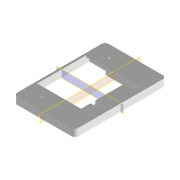
# Autodesk Inventor part: TIRFImager_base_v0
Saved by Autodesk Inventor 2022 (Build 260153000, 153)
## iProperties
Created: 2022-05-21
Part Number: TIRFImager_base_v0
Material: Generisch
Document SubType Name: Modeling
Designer: diederichbenedict
Density: 1 g/cm^3
Appearance: Vorgabe
Author: diederichbenedict
Autodesk Inventor part; units mm, degrees
ref_plane "YZ Plane" through (0, 0, 0) normal (1, 0, 0) x (0, 1, 0)
ref_plane "XZ Plane" through (0, 0, 0) normal (0, 1, 0) x (-1, 0, 0)
ref_plane "XY Plane" through (0, 0, 0) normal (0, 0, 1) x (1, 0, 0)
sketch "Skizze1" plane through (0, 0, 0) normal (0, 1, 0) x (-1, 0, 0)
  line L0 (-37.75, -63.9) -> (37.75, -63.9)
  line L1 (42.75, -58.9) -> (42.75, 58.9)
  line L2 (37.75, 63.9) -> (-37.75, 63.9)
  line L3 (-42.75, 58.9) -> (-42.75, -58.9)
  line L4 (-42.75, -63.9) -> (42.75, 63.9) construction
  line L5 (42.75, -63.9) -> (-42.75, 63.9) construction
  arc A0 (42.75, 58.9) -> (37.75, 63.9) centre (37.75, 58.9) ccw
  arc A1 (-37.75, 63.9) -> (-42.75, 58.9) centre (-37.75, 58.9) ccw
  arc A2 (-42.75, -58.9) -> (-37.75, -63.9) centre (-37.75, -58.9) ccw
  arc A3 (37.75, -63.9) -> (42.75, -58.9) centre (37.75, -58.9) ccw
  point P0 (0, 0)
  dimension "d0" = 85.5
  dimension "d1" = 127.8
  dimension "d2" = 5
  constraints: 12 end point, 8 point on circle, 8 point on line, 8 tangent, 4 centre point, 3 equal radius, 2 midpoint, 2 parallel, 1 horizontal, 1 perpendicular
  measures "d0" distance of L5.end L4.end
  measures "d1" distance of L4.end L5.start
  measures "d2" radius of A0
extrude "Extrusion1" add sketch "Skizze1" along normal blind 10
ref_plane "Arbeitsebene1" through (37.75, 0, 0) normal (0, 0, -1) x (-1, 0, 0)
ref_plane "Arbeitsebene2" through (0, 0, 58.9) normal (1, 0, 0) x (0, 0, -1)
sketch "Skizze2" plane through (0, 10, 0) normal (0, 1, 0) x (1, 0, 0)
  line L0 (-12.95, 38) -> (-38.75, 38) projected
  line L1 (-38.75, -38) -> (-12.95, -38) projected
  line L2 (-12.95, -38) -> (-12.95, -2.5) projected
  line L3 (-38.75, 38) -> (-38.75, -38) projected
  line L4 (-38.75, -38) -> (-12.95, -38)
  line L5 (-12.95, -38) -> (-12.95, 38)
  line L6 (-12.95, 38) -> (-38.75, 38)
  line L7 (-38.75, 38) -> (-38.75, -38)
  line L8 (-11.95, 39) -> (-11.95, -39)
  line L9 (-11.95, -39) -> (-39.75, -39)
  line L10 (-39.75, -39) -> (-39.75, 39)
  line L11 (-39.75, 39) -> (-11.95, 39)
  point P0 (0, 0)
  dimension "d5" = 1
  constraints: 16 end point, 4 parallel, 2 perpendicular, 1 horizontal, 3 other
  measures "d5" distance between parallel lines of L5 L8
extrude "Extrusion2" cut sketch "Skizze2" against normal through all contours L5 L2 L1 L3 L0 | L8 L9 L10 L11
ref_plane "Arbeitsebene3" through (-32.75, 5, -38) normal (0, 1, 0) x (0, 0, 1)
sketch "Skizze3" plane through (0, 10, 0) normal (0, 1, 0) x (1, 0, 0)
  line L0 (-11.95, -39) -> (-39.75, -39) projected
  line L1 (-39.75, -39) -> (-39.75, 39) projected
  line L2 (-39.75, 39) -> (-11.95, 39) projected
  line L3 (-11.95, 39) -> (-11.95, -39) projected
  arc A0 (-37.75, 63.9) -> (-42.75, 58.9) centre (-37.75, 58.9) ccw projected
  line L4 (-42.75, 58.9) -> (-42.75, -58.9) projected
  arc A1 (-42.75, -58.9) -> (-37.75, -63.9) centre (-37.75, -58.9) ccw projected
  line L5 (-37.75, -63.9) -> (37.75, -63.9) projected
  arc A2 (37.75, -63.9) -> (42.75, -58.9) centre (37.75, -58.9) ccw projected
  line L6 (42.75, -58.9) -> (42.75, 58.9) projected
  arc A3 (42.75, 58.9) -> (37.75, 63.9) centre (37.75, 58.9) ccw projected
  line L7 (37.75, 63.9) -> (-37.75, 63.9) projected
  line L8 (-39.75, -39) -> (-39.75, 39) projected
  line L9 (-11.95, 39) -> (-11.95, -39) projected
  line L10 (-39.75, -39) -> (-11.95, -39)
  line L11 (-11.95, -39) -> (-11.95, -34)
  line L12 (-11.95, -34) -> (-39.75, -34)
  line L13 (-39.75, -34) -> (-39.75, -39)
  line L14 (-39.75, 39) -> (-11.95, 39)
  line L15 (-11.95, 39) -> (-11.95, 34)
  line L16 (-11.95, 34) -> (-39.75, 34)
  line L17 (-39.75, 34) -> (-39.75, 39)
  point P0 (0, 0)
  point P1 (-11.95, -34)
  dimension "d8" = 27.8
  dimension "d9" = 5
  dimension "d10" = 5
  constraints: 16 end point, 4 parallel, 2 horizontal, 2 perpendicular, 2 point on line
  measures "d8" distance of L12.end L11.end
  measures "d9" distance of L11.end L10.end
  measures "d10" distance of L14.end L15.end
extrude "Extrusion3" add sketch "Skizze3" against normal blind 1 contours L0 L1 L12 L3 | L16 L1 L2 L3
sketch "Skizze4" plane through (0, 0, 0) normal (0, -1, 0) x (1, 0, 0)
  line L0 (-39.75, 39) -> (-11.95, 39) projected
  line L1 (-11.95, 39) -> (-11.95, -39) projected
  line L2 (-11.95, -39) -> (-39.75, -39) projected
  line L3 (-39.75, -39) -> (-39.75, 39) projected
  arc A0 (-42.75, -58.9) -> (-37.75, -63.9) centre (-37.75, -58.9) ccw projected
  line L4 (37.75, -63.9) -> (-37.75, -63.9) projected
  arc A1 (37.75, -63.9) -> (42.75, -58.9) centre (37.75, -58.9) ccw projected
  line L5 (42.75, 58.9) -> (42.75, -58.9) projected
  arc A2 (42.75, 58.9) -> (37.75, 63.9) centre (37.75, 58.9) ccw projected
  line L6 (-37.75, 63.9) -> (37.75, 63.9) projected
  arc A3 (-37.75, 63.9) -> (-42.75, 58.9) centre (-37.75, 58.9) ccw projected
  line L7 (-42.75, -58.9) -> (-42.75, 58.9) projected
  line L8 (-11.95, -34) -> (-11.95, 34) projected
  line L9 (-11.95, 34) -> (12.75, 34)
  line L10 (12.75, 34) -> (12.75, -34)
  line L11 (12.75, -34) -> (-11.95, -34)
  line L12 (-11.95, -34) -> (-11.95, 34)
  line L13 (-2.45, 7.5) -> (-2.45, -8) projected
  line L14 (12.75, -34.1) -> (12.75, -39.1) projected
  point P0 (0, 0)
  point P1 (-11.95, -34)
  dimension "d14" = 5
  dimension "d15" = 5
  dimension "d44" = 0
  constraints: 8 end point, 2 parallel, 1 horizontal, 1 perpendicular, 1 point on line
  measures "d14" distance between parallel lines of L2 L11
  measures "d15" distance between parallel lines of L9 L0
  measures "d44" distance between parallel lines of L14 L10
extrude "Extrusion4" cut sketch "Skizze4" against normal through all contours L9 L10 L11 L1
sketch "Skizze5" plane through (0, 0, 0) normal (0, -1, 0) x (1, 0, 0)
  arc A0 (-42.75, -58.9) -> (-37.75, -63.9) centre (-37.75, -58.9) ccw projected
  line L0 (37.75, -63.9) -> (-37.75, -63.9) projected
  arc A1 (37.75, -63.9) -> (42.75, -58.9) centre (37.75, -58.9) ccw projected
  line L1 (42.75, 58.9) -> (42.75, -58.9) projected
  arc A2 (42.75, 58.9) -> (37.75, 63.9) centre (37.75, 58.9) ccw projected
  line L2 (-37.75, 63.9) -> (37.75, 63.9) projected
  arc A3 (-37.75, 63.9) -> (-42.75, 58.9) centre (-37.75, 58.9) ccw projected
  line L3 (-42.75, -58.9) -> (-42.75, 58.9) projected
  line L4 (-11.95, 34) -> (12.75, 34) projected
  line L5 (12.75, 34) -> (12.75, -34) projected
  line L6 (12.75, -34) -> (-11.95, -34) projected
  line L7 (-11.95, -34) -> (-11.95, -39) projected
  line L8 (-11.95, -39) -> (-39.75, -39) projected
  line L9 (-39.75, -39) -> (-39.75, 39) projected
  line L10 (-39.75, 39) -> (-11.95, 39) projected
  line L11 (-11.95, 39) -> (-11.95, 34) projected
  circle A4 centre (-19.85, -47) radius 1.4
  circle A5 centre (-19.85, 47) radius 1.4
  point P0 (0, 0)
  dimension "d18" = 2.8
  dimension "d19" = 2.8
  dimension "d20" = 8
  dimension "d21" = 8
  constraints: 2 centre point
  measures "d18" diameter of A4
  measures "d19" diameter of A5
  measures "d20" distance from line of L8 A4.centre
  measures "d21" distance from line of A5.centre L10
extrude "Extrusion5" cut sketch "Skizze5" against normal through all contours A4 | A5
sketch "Skizze9" plane through (0, 9, 0) normal (0, -1, 0) x (1, 0, 0)
  circle A0 centre (-19.85, 47) radius 1.4 projected
  circle A1 centre (-19.85, -47) radius 1.4 projected
  arc A2 (-42.75, -58.9) -> (-37.75, -63.9) centre (-37.75, -58.9) ccw projected
  line L0 (37.75, -63.9) -> (-37.75, -63.9) projected
  arc A3 (37.75, -63.9) -> (42.75, -58.9) centre (37.75, -58.9) ccw projected
  line L1 (42.75, 58.9) -> (42.75, -58.9) projected
  arc A4 (42.75, 58.9) -> (37.75, 63.9) centre (37.75, 58.9) ccw projected
  line L2 (-37.75, 63.9) -> (37.75, 63.9) projected
  arc A5 (-37.75, 63.9) -> (-42.75, 58.9) centre (-37.75, 58.9) ccw projected
  line L3 (-42.75, -58.9) -> (-42.75, 58.9) projected
  line L4 (12.75, 34) -> (12.75, -34) projected
  line L5 (12.75, -34) -> (-11.95, -34) projected
  line L6 (-11.95, -34) -> (-11.95, -39) projected
  line L7 (-11.95, -39) -> (-39.75, -39) projected
  line L8 (-39.75, -39) -> (-39.75, 39) projected
  line L9 (-39.75, 39) -> (-11.95, 39) projected
  line L10 (-11.95, 39) -> (-11.95, 34) projected
  line L11 (-11.95, 34) -> (12.75, 34) projected
  line L12 (-39.75, 39) -> (-11.95, 39) projected
  line L13 (-39.75, 39) -> (-11.95, 39)
  line L14 (-11.95, 39) -> (-11.95, 34)
  line L15 (-11.95, 34) -> (-39.75, 34)
  line L16 (-39.75, 34) -> (-39.75, 39)
  line L17 (-11.95, -39) -> (-39.75, -39) projected
  line L18 (-39.75, -39) -> (-39.75, -34) projected
  line L19 (-11.95, -39) -> (-39.75, -39)
  line L20 (-39.75, -39) -> (-39.75, -34)
  line L21 (-39.75, -34) -> (-11.95, -34)
  line L22 (-11.95, -34) -> (-11.95, -39)
  point P0 (0, 0)
  point P1 (-11.95, -34)
  constraints: 16 end point, 4 parallel, 2 horizontal, 2 perpendicular
extrude "Extrusion8" add sketch "Skizze9" along normal blind 1 contours L15 L8 L9 L10 | L6 L7 L8 L21
sketch "Skizze10" plane through (0, 10, 0) normal (0, 1, 0) x (1, 0, 0)
  line L0 (23.25, -52.9) -> (23.25, 33.1) projected
  line L1 (23.25, -52.9) -> (14.45, -52.9) projected
  line L2 (14.45, -52.9) -> (14.45, 33.1) projected
  line L3 (14.45, 33.1) -> (23.25, 33.1) projected
  circle A0 centre (19.25, -37.4) radius 3.25 projected
  circle A1 centre (19.25, 17.6) radius 3.25 projected
  line L4 (41.05, -52.9) -> (41.05, 33.1) projected
  line L5 (41.05, -52.9) -> (32.25, -52.9) projected
  line L6 (32.25, -52.9) -> (32.25, 33.1) projected
  line L7 (32.25, 33.1) -> (41.05, 33.1) projected
  circle A2 centre (36.25, -37.4) radius 3.25 projected
  circle A3 centre (36.25, 17.6) radius 3.25 projected
  point P0 (0, 0)
hole "Bohrung2" at (36.25, 10, 37.4) at (36.25, 10, -17.6) at (19.25, 10, 37.4) at (19.25, 10, -17.6) direction (0, -1, 0) diameter 2.8 end through all counterbore diameter 6.5 counterbore depth 4
